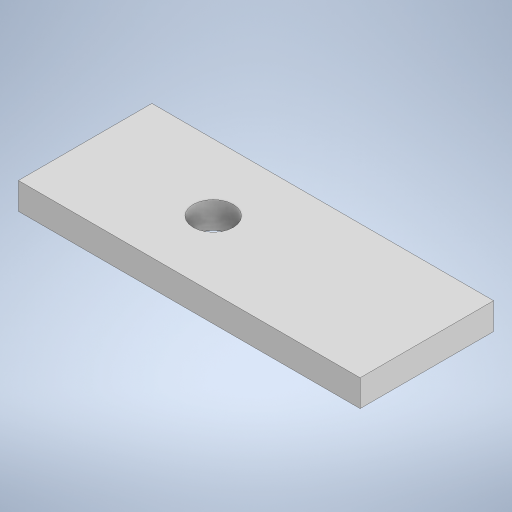
# Autodesk Inventor part: Part3 x 2
Saved by Autodesk Inventor 2023.1 (Build 271208000, 208)
## iProperties
Created: 2022-10-24
Part Number: Part3 x 2
Material: Generic
Document SubType Name: Modeling
Designer: jshin23
Density: 1 g/cm^3
Appearance: Default
Author: jshin23
Autodesk Inventor part; units mm, degrees
ref_plane "YZ Plane" through (0, 0, 0) normal (1, 0, 0) x (0, 1, 0)
ref_plane "XZ Plane" through (0, 0, 0) normal (0, 1, 0) x (-1, 0, 0)
ref_plane "XY Plane" through (0, 0, 0) normal (0, 0, 1) x (1, 0, 0)
sketch "Sketch1" plane through (0, 0, 0) normal (0, 1, 0) x (-1, 0, 0)
  line L0 (0, 31.75) -> (162.56, 31.75)
  line L1 (162.56, 31.75) -> (162.56, -31.75)
  line L2 (162.56, -31.75) -> (0, -31.75)
  line L3 (0, -31.75) -> (0, 31.75)
  circle A0 centre (101.6, 0) radius 9.525
  point P0 (0, 0)
  point P1 (0, 0)
  dimension "d0" = 162.56
  dimension "d1" = 63.5
  dimension "d5" = 19.05
  dimension "d6" = 60.96
  dimension "d7" = 31.75
  constraints: 8 end point, 2 parallel, 1 centre point, 1 coincident, 1 horizontal, 1 midpoint, 1 perpendicular
  measures "d0" distance of L1.end L2.end
  measures "d1" distance of L2.end L0.start
  measures "d5" diameter of A0
  measures "d6" distance from line of L1 A0.centre
  measures "d7" distance from line of L2 A0.centre
extrude "Extrusion1" add sketch "Sketch1" along normal blind 12.7
body "Solid1"
